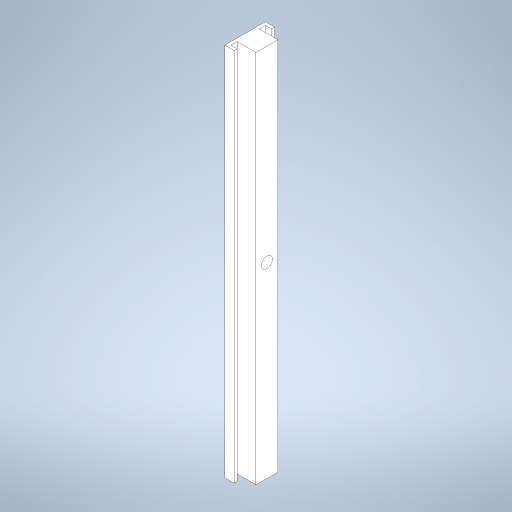
# Autodesk Inventor part: Stringer cap
Saved by Autodesk Inventor 2024 (Build 280153000, 153)
## iProperties
Created: 2024-05-14
Part Number: Stringer cap
Material: Generic
Document SubType Name: Modeling
Designer: auror
Density: 1 g/cm^3
Appearance: Default
Author: auror
Autodesk Inventor part; units mm, degrees
ref_plane "YZ Plane" through (0, 0, 0) normal (1, 0, 0) x (0, 1, 0)
ref_plane "XZ Plane" through (0, 0, 0) normal (0, 1, 0) x (-1, 0, 0)
ref_plane "XY Plane" through (0, 0, 0) normal (0, 0, 1) x (1, 0, 0)
sketch "Sketch1" plane through (0, 0, 0) normal (0, 1, 0) x (-1, 0, 0)
  line L0 (3.5, 3.5) -> (-2.5, 3.5)
  line L1 (-2.5, 3.5) -> (-2.5, -3.5)
  line L2 (-2.5, -3.5) -> (3.5, -3.5)
  line L3 (4.5, -3.5) -> (4.5, 3.5)
  line L4 (4.5, 3.5) -> (4.5, 6.5)
  line L5 (4.5, 6.5) -> (1.5, 6.5)
  line L6 (1.5, 6.5) -> (1.5, 5.5)
  line L7 (1.5, 5.5) -> (3.5, 5.5)
  line L8 (3.5, 5.5) -> (3.5, 3.5)
  line L9 (4.5, -3.5) -> (4.5, -6.5)
  line L10 (4.5, -6.5) -> (1.5, -6.5)
  line L11 (1.5, -6.5) -> (1.5, -5.5)
  line L12 (1.5, -5.5) -> (3.5, -5.5)
  line L13 (3.5, -5.5) -> (3.5, -3.5)
  point P0 (0, 0)
  dimension "d2" = 3.5
  dimension "d3" = 4.5
  dimension "d4" = 1
  dimension "d5" = 1
  dimension "d6" = 2
  dimension "d7" = 2
  dimension "d8" = 7
  dimension "d9" = 7
  dimension "d10" = 1
  dimension "d11" = 1
  dimension "d12" = 3
  dimension "d13" = 3
  constraints: 28 end point, 6 perpendicular, 5 parallel, 2 collinear, 1 horizontal
  measures "d2" distance from line of point (0, 0) L0
  measures "d3" distance from line of point (0, 0) L3
  measures "d4" distance between parallel lines of L8 L4
  measures "d5" distance between parallel lines of L13 L9
  measures "d6" distance between parallel lines of L7 L0
  measures "d7" distance between parallel lines of L12 L2
  measures "d8" distance between parallel lines of L1 L3
  measures "d9" distance between parallel lines of L2 L0
  measures "d10" distance between parallel lines of L7 L5
  measures "d11" distance between parallel lines of L10 L12
  measures "d12" distance between parallel lines of L6 L4
  measures "d13" distance between parallel lines of L11 L9
extrude "Extrusion1" add sketch "Sketch1" along normal blind 120
sketch "Sketch2" plane through (-4.5, 0, -6.5) normal (-1, 0, 0) x (0, 0, 1)
  line L0 (0, 0) -> (13, 0) projected
  line L1 (0, 0) -> (0, 120) projected
  point P0 (6.5, 0)
  point P1 (6.5, 60)
  dimension "d16" = 60
  dimension "d17" = 6.5
  measures "d16" distance from line of L0 point (6.5, 60)
  measures "d17" distance from line of point (6.5, 60) L1
hole "Hole1" at (-4.5, 60, 0) direction (1, 0, 0) diameter 3.5 end through all
body "Solid1"
